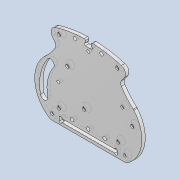
# Autodesk Inventor part: 脚中間フレーム内v2
Saved by Autodesk Inventor 2020 (Build 240168000, 168)
## iProperties
Created: 2021-02-23
Part Number: 脚中間フレーム内v2
Material: アルミニウム 2014-T4
Document SubType Name: Modeling
Designer: AA19065
Density: 2.8 g/cm^3
Appearance: サテン
Author: AA19065
Autodesk Inventor part; units mm, degrees
ref_plane "YZ Plane" through (0, 0, 0) normal (1, 0, 0) x (0, 1, 0)
ref_plane "XZ Plane" through (0, 0, 0) normal (0, 1, 0) x (-1, 0, 0)
ref_plane "XY Plane" through (0, 0, 0) normal (0, 0, 1) x (1, 0, 0)
sketch "スケッチ1" plane through (0, 0, 0) normal (0, 0, 1) x (1, 0, 0)
  circle A0 centre (70, 10) radius 6.025 construction
  line L0 (-57.99, -53) -> (89.5137, -53) construction
  line L1 (-38.7488, -33) -> (132.6572, -33) construction
  circle A1 centre (0, 20) radius 9 construction
  circle A2 centre (76.6032, -15) radius 10.2409 construction
  circle A3 centre (78.6778, 20) radius 3 construction
  circle A4 centre (78.6778, 20) radius 1.25 construction
  circle A5 centre (76.6032, -15) radius 1.25
  arc A6 (7.8087, -33.9687) -> (78.0973, 6.0713) centre (13.7692, 37.2822) ccw construction
  line L2 (108, 72.8318) -> (108, -27.6373) construction
  circle A7 centre (146, 10) radius 6.025 construction
  line L3 (273.99, -53) -> (126.4863, -53) construction
  arc A8 (78.4128, 35.7709) -> (77.7684, 14.5445) centre (95.0314, 24.6434) ccw construction
  arc A9 (66.9642, -15.6785) -> (76.6032, -15) centre (70, 10) ccw construction
  circle A10 centre (66.9642, -15.6785) radius 10.2409 construction
  arc A11 (-3.9904, -8.067) -> (76.0896, 3.373) centre (27.7113, 56.0206) ccw construction
  circle A12 centre (78.6778, 20) radius 9.0064 construction
  circle A13 centre (76.6032, -15) radius 5
  arc A14 (73.3391, 27.2536) -> (73.703, -19.0729) centre (90.2907, 4.222) ccw
  circle A15 centre (70, 10) radius 1.5
  circle A16 centre (70, 10) radius 3 construction
  circle A17 centre (70, 10) radius 7.5 construction
  line L4 (254.7488, -33) -> (83.3428, -33) construction
  circle A18 centre (139.3968, -15) radius 10.2409 construction
  circle A19 centre (139.3968, -15) radius 1.25
  circle A20 centre (139.3968, -15) radius 5
  circle A21 centre (149.0358, -15.6785) radius 10.2409 construction
  arc A22 (139.9104, 3.373) -> (219.9904, -8.067) centre (188.2887, 56.0206) ccw construction
  arc A23 (137.9027, 6.0713) -> (208.1913, -33.9687) centre (202.2308, 37.2822) ccw construction
  arc A24 (139.3968, -15) -> (149.0358, -15.6785) centre (146, 10) ccw construction
  circle A25 centre (146, 10) radius 1.5
  circle A26 centre (146, 10) radius 3 construction
  arc A27 (142.297, -19.0729) -> (142.6609, 27.2536) centre (125.7093, 4.222) ccw
  circle A28 centre (137.3222, 20) radius 1.25
  circle A29 centre (137.3222, 20) radius 3 construction
  circle A30 centre (146, 10) radius 7.5 construction
  circle A31 centre (137.3222, 20) radius 9.0064
  arc A32 (138.2316, 14.5445) -> (137.5872, 35.7709) centre (120.9686, 24.6434) ccw construction
  circle A33 centre (146, 10) radius 6.025 construction
  line L5 (76.6032, -20) -> (139.3968, -20)
  circle A34 centre (75.92, 37.44) radius 3 construction
  arc A35 (36.1592, 11.7228) -> (78.4714, 35.8619) centre (35.1383, 62.6652) ccw construction
  arc A36 (78.3972, 39.1322) -> (46.2745, 63.7904) centre (24.7284, 2.4693) ccw construction
  arc A37 (79.2229, 39.6963) -> (48.1614, 64.1653) centre (24.7284, 2.4693) ccw
  arc A38 (35.9338, 10.7187) -> (79.3218, 35.3358) centre (35.1383, 62.6652) ccw
  circle A39 centre (75.92, 37.44) radius 4
  arc A40 (75.2035, 49.567) -> (74.2797, 46.0602) centre (75.92, 47.5032) ccw
  arc A41 (32.1622, 54.9956) -> (-29.3454, 24.6971) centre (28.3773, -14.902) ccw construction
  line L6 (75.92, 47.5032) -> (75.92, 37.44) construction
  circle A42 centre (140.08, 37.44) radius 3 construction
  circle A43 centre (140.08, 37.44) radius 4
  line L7 (140.08, 47.5032) -> (140.08, 37.44) construction
  arc A44 (169.7255, 63.7904) -> (137.6028, 39.1322) centre (191.2716, 2.4693) ccw construction
  arc A45 (167.8386, 64.1653) -> (136.7771, 39.6963) centre (191.2716, 2.4693) ccw
  arc A46 (141.7203, 46.0602) -> (140.7965, 49.567) centre (140.08, 47.5032) ccw
  arc A47 (137.5286, 35.8619) -> (179.8408, 11.7228) centre (180.8617, 62.6652) ccw construction
  arc A48 (136.6782, 35.3358) -> (180.0662, 10.7187) centre (180.8617, 62.6652) ccw
  arc A49 (138.2316, 14.5445) -> (137.5872, 35.7709) centre (120.9686, 24.6434) ccw construction
  line L8 (78.6778, 20) -> (76.6032, -15) construction
  arc A50 (140.7965, 49.567) -> (75.2035, 49.567) centre (108, -44.902) ccw
  line L9 (9.726, 55.098) -> (56.6721, 55.098) construction
  line L10 (83, -14.5) -> (133, -14.5)
  line L11 (133, -14.5) -> (133, -17.5)
  line L12 (133, -17.5) -> (83, -17.5)
  line L13 (83, -17.5) -> (83, -14.5)
  arc A51 (83, -17.5) -> (85.1, -17.5) centre (84.05, -17.5) ccw
  line L14 (83, -17.5) -> (84.05, -17.5) construction
  line L15 (85.1, -17.5) -> (84.05, -17.5) construction
  arc A52 (85.1, -14.5) -> (83, -14.5) centre (84.05, -14.5) ccw
  line L16 (83, -14.5) -> (84.05, -14.5) construction
  line L17 (85.1, -14.5) -> (84.05, -14.5) construction
  arc A53 (133, -14.5) -> (130.9, -14.5) centre (131.95, -14.5) ccw
  line L18 (133, -14.5) -> (131.95, -14.5) construction
  line L19 (130.9, -14.5) -> (131.95, -14.5) construction
  arc A54 (130.9, -17.5) -> (133, -17.5) centre (131.95, -17.5) ccw
  line L20 (133, -17.5) -> (131.95, -17.5) construction
  line L21 (130.9, -17.5) -> (131.95, -17.5) construction
  circle A55 centre (94, -11) radius 1.5
  circle A56 centre (108, -11) radius 1.5
  circle A57 centre (122, -11) radius 1.5
  circle A58 centre (82.5564, 47.1333) radius 3
  circle A59 centre (133, 47.1333) radius 3
  circle A60 centre (82.5, -8) radius 3
  circle A61 centre (133.5, -8) radius 3
  circle A62 centre (82.5564, 47.1333) radius 1.5
  circle A63 centre (133, 47.1333) radius 1.5
  circle A64 centre (133.5, -8) radius 1.5
  circle A65 centre (82.5, -8) radius 1.5
  line L22 (93.8618, 55.098) -> (128.6737, 55.098) construction
  circle A66 centre (96.5938, 51) radius 1.5
  circle A67 centre (119.4062, 51) radius 1.5
  line L23 (105.5, 57.098) -> (110.5, 57.098)
  line L24 (110.5, 57.098) -> (110.5, 50.098)
  line L25 (110.5, 50.098) -> (105.5, 50.098)
  line L26 (105.5, 50.098) -> (105.5, 57.098)
  line L27 (82.5564, 47.1333) -> (104.0735, 2) construction
  circle A68 centre (82.5564, 47.1333) radius 3
  circle A69 centre (82.5564, 47.1333) radius 1.5
  circle A70 centre (104.0735, 2) radius 6.025
  circle A71 centre (104.0735, 2) radius 1.5
  line L28 (82.5564, 47.1333) -> (48.483, 55.1333) construction
  line L29 (48.483, 55.1333) -> (70, 10) construction
  line L30 (70, 10) -> (104.0735, 2) construction
  line L31 (82.5564, 47.1333) -> (53.8336, 67.1333) construction
  line L32 (53.8336, 67.1333) -> (75.3506, 22) construction
  line L33 (75.3506, 22) -> (104.0735, 2) construction
  line L34 (82.5564, 47.1333) -> (48.2636, 40.1333) construction
  line L35 (48.2636, 40.1333) -> (69.7806, -5) construction
  line L36 (69.7806, -5) -> (104.0735, 2) construction
  line L37 (48.483, 55.1333) -> (82.5564, 47.1333) construction
  circle A72 centre (76.6032, -15) radius 3
  arc A73 (-4.2099, -23.067) -> (75.8702, -11.627) centre (27.4919, 41.0206) ccw construction
  arc A74 (75.3506, 22) -> (69.7806, -5) centre (104.0735, 2) ccw construction
  arc A75 (72.7246, 23.8286) -> (66.6452, -5.64) centre (104.0735, 2) ccw
  arc A76 (77.9767, 20.1714) -> (72.9159, -4.36) centre (104.0735, 2) ccw
  arc A77 (77.9767, 20.1714) -> (72.7246, 23.8286) centre (75.3506, 22) ccw
  arc A78 (66.6452, -5.64) -> (72.9159, -4.36) centre (69.7806, -5) ccw
  line L38 (70, 10) -> (84.8776, 23.3663) construction
  line L39 (84.8776, 23.3663) -> (104.0735, 2) construction
  line L40 (81.126, 7.3878) -> (84.8776, 23.3663) construction
  circle A79 centre (82.0403, 11.2819) radius 1.25
  arc A80 (79.4181, 50.9264) -> (76.8573, 42.9425) centre (80.8701, 46.058) ccw
  arc A81 (139.1427, 42.9425) -> (136.5819, 50.9264) centre (135.1299, 46.058) ccw
  arc A82 (136.5819, 50.9264) -> (79.4181, 50.9264) centre (108, -44.902) ccw
  line L41 (82.5564, 47.1333) -> (104.0735, 2) construction
  circle A83 centre (90, 27) radius 3
  circle A84 centre (90, 27) radius 1.5
  line L42 (108, 72.8994) -> (108, -27.2053) construction
  line L43 (110.5, 57.098) -> (110.5, 50.098)
  line L44 (110.5, 50.098) -> (105.5, 50.098)
  line L45 (105.5, 50.098) -> (105.5, 57.098)
  arc A85 (105.5, 52.198) -> (105.5, 50.098) centre (105.5, 51.148) ccw
  line L46 (105.5, 50.098) -> (105.5, 51.148) construction
  line L47 (105.5, 52.198) -> (105.5, 51.148) construction
  arc A86 (110.5, 50.098) -> (110.5, 52.198) centre (110.5, 51.148) ccw
  line L48 (110.5, 50.098) -> (110.5, 51.148) construction
  line L49 (110.5, 52.198) -> (110.5, 51.148) construction
  line L50 (105.5, 57.098) -> (105.5, 44.098)
  line L51 (105.5, 44.098) -> (110.5, 44.098)
  line L52 (110.5, 44.098) -> (110.5, 57.098)
  circle A87 centre (108, 47.098) radius 1.25
  point P0 (0, 0)
  point P1 (0, 0)
  point P2 (81.3036, 36.7164)
  point P3 (76.9481, 1.1491)
  point P4 (139.0519, 1.1491)
  point P5 (134.6964, 36.7164)
  point P6 (108, -14.5)
  point P7 (108, 57.098)
  point P8 (105.5, 55.0668)
  point P9 (68.8141, 23.1049)
  point P10 (147.1859, 23.1049)
  point P11 (143.7549, 26.3036)
  point P12 (143.3172, 26.7558)
  point P13 (136.6782, 35.3358)
  point P14 (136.7771, 39.6963)
  point P15 (110.5, 55.0668)
  point P16 (85.1, -17.5)
  point P17 (130.9, -14.5)
  point P18 (76.0326, 47.6096)
  point P19 (79.4181, 50.9264)
  point P20 (76.8573, 42.9425)
  point P21 (136.5819, 50.9264)
  point P22 (108, -14.1156)
  point P23 (108, -10.6283)
  point P24 (108, 57.098)
  dimension "d0" = 53
  dimension "d1" = 6
  dimension "d2" = 2.5
  dimension "d3" = 2.5
  dimension "d4" = 15
  dimension "d5" = 76
  dimension "d6" = 20
  dimension "d7" = 25.8573
  dimension "d8" = 10
  dimension "d9" = 3
  dimension "d10" = 6
  dimension "d11" = 15
  dimension "d12" = 1
  dimension "d13" = 1
  dimension "d14" = 1
  dimension "d15" = 100
  dimension "d16" = 50
  dimension "d17" = 3
  dimension "d18" = 1.05
  dimension "d19" = 180
  dimension "d20" = 1.05
  dimension "d21" = 180
  dimension "d22" = 1.05
  dimension "d23" = 180
  dimension "d24" = 1.05
  dimension "d25" = 180
  dimension "d26" = 3
  dimension "d27" = 3
  dimension "d28" = 3
  dimension "d29" = 14
  dimension "d30" = 14
  dimension "d31" = 3.5
  dimension "d32" = 2.5
  dimension "d33" = 6
  dimension "d34" = 6
  dimension "d35" = 6
  dimension "d36" = 6
  dimension "d37" = 3
  dimension "d38" = 3
  dimension "d39" = 3
  dimension "d40" = 3
  dimension "d41" = 25.5
  dimension "d42" = 25.5
  dimension "d43" = 12
  dimension "d44" = 25
  dimension "d45" = 3
  dimension "d46" = 2
  dimension "d47" = 7
  dimension "d48" = 5
  dimension "d49" = 6
  dimension "d50" = 3
  dimension "d51" = 12.05
  dimension "d52" = 3
  dimension "d53" = 35
  dimension "d54" = 12
  dimension "d55" = 15
  dimension "d56" = 33
  dimension "d57" = 35.5
  dimension "d58" = 6
  dimension "d59" = 6.4
  dimension "d60" = 20
  dimension "d61" = 2.5
  dimension "d62" = 4
  dimension "d72" = 100
  constraints: 106 end point, 86 point on circle, 84 centre point, 47 symmetric about line, 29 coincident, 24 tangent, 12 parallel, 12 point on line, 7 horizontal, 6 vertical, 4 horizontal alignment, 4 perpendicular, 2 equal length, 2 midpoint, 1 concentric, 1 equal radius, 53 other
  measures "d0" distance from line of L1 A1.centre
  measures "d1" diameter of A3
  measures "d2" diameter of A4
  measures "d3" diameter of A5
  measures "d4" vertical distance of point (0, 0) A2.centre
  measures "d5" distance of A7.centre A0.centre
  measures "d6" vertical distance of point (0, 0) A3.centre
  measures "d7" distance of A2.centre A0.centre
  measures "d8" diameter of A13
  measures "d9" diameter of A15
  measures "d10" diameter of A16
  measures "d11" diameter of A17
  measures "d12" radial gap between concentric circles of A36 A37
  measures "d13" radial gap between concentric circles of A35 A38
  measures "d15" radius of A50
  measures "d16" distance of L11.end L12.end
  measures "d17" distance of L10.end L11.end
  measures "d18" radius of A51
  measures "d19" angle of L14 L15
  measures "d20" radius of A52
  measures "d21" angle of L16 L17
  measures "d22" radius of A53
  measures "d23" angle of L18 L19
  measures "d24" radius of A54
  measures "d25" angle of L20 L21
  measures "d26" diameter of A55
  measures "d27" diameter of A56
  measures "d28" diameter of A57
  measures "d29" distance of A55.centre A56.centre
  measures "d30" distance of A57.centre A56.centre
  measures "d31" distance from line of L10 A56.centre
  measures "d32" distance between parallel lines of L5 L12
  measures "d33" diameter of A58
  measures "d34" diameter of A59
  measures "d35" diameter of A60
  measures "d36" diameter of A61
  measures "d37" diameter of A62
  measures "d38" diameter of A63
  measures "d39" diameter of A64
  measures "d40" diameter of A65
  measures "d41" distance from line of L2 A65.centre
  measures "d42" distance from line of A64.centre L2
  measures "d43" distance from line of A65.centre L5
  measures "d44" distance from line of A63.centre L2
  measures "d45" diameter of A66
  measures "d46" distance between parallel lines of L22 L23
  measures "d47" distance between parallel lines of L25 L23
  measures "d48" distance between parallel lines of L24 L26
  measures "d49" diameter of A68
  measures "d50" diameter of A69
  measures "d51" diameter of A70
  measures "d52" diameter of A71
  measures "d53" distance of L28.start L28.end
  measures "d54" vertical distance of L31.end L28.end
  measures "d55" vertical distance of L34.end L28.end
  measures "d56" distance between parallel lines of L0 L5
  measures "d57" distance between parallel lines of L0 L12
  measures "d58" diameter of A72
  measures "d59" diameter of A77
  measures "d60" distance of L29.end L38.end
  measures "d61" diameter of A79
  measures "d62" distance from line of L30 A79.centre
  measures "d72" radius of A82
extrude "押し出し1" add sketch "スケッチ1" along normal blind 3 contours A13 | A13 A14 A38 A39 A37 A80 A50 L26 A85 L50 L51 L52 A86 L24 A81 A45 A43 A48 A27 A31 A20 L5 | A20 | A48 A31 A27 | A31 | L25 L52 L51 L50 | A58 | A59 | A60 | A61 | A70 | A72 | A83
fillet "フィレット1" radius 1.05 2 edges at (105.5, 55.0668, 1.5) (110.5, 55.0668, 1.5)
fillet "フィレット2" radius 5 2 edges at (68.8141, 23.1049, 1.5) (147.1859, 23.1049, 1.5)
chamfer "面取り2" distance 2 angle 45 10 edges at (131.5, 47.1333, 0) (81.0564, 47.1333, 0) (88.5, 27, 0) (102.5735, 2, 0) (81, -8, 0) (75.3532, -15, 0) (138.1468, -15, 0) (144.5, 10, 0) (136.0722, 20, 0) (132, -8, 0)
equation "\"d0\" = d63"
equation "\"d20\" = d18"
equation "\"d22\" = d24"
equation "\"d24\" = d18"
equation "\"d30\" = d29"
equation "\"d42\" = d41"
equation "\"d44\" = d64"
equation "\"d53\" = d65"
equation "\"d54\" = d66"
equation "\"d55\" = d67"
equation "\"d63\" = 53"
equation "\"d64\" = 25"
equation "\"d65\" = 35"
equation "\"d66\" = 12"
equation "\"d67\" = 15"
